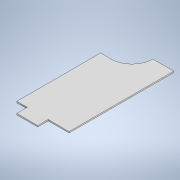
# Autodesk Inventor part: Rotation Board
Saved by Autodesk Inventor 2020 (Build 240168000, 168)
## iProperties
Created: 2021-02-27
Part Number: Rotation Board
Material: Generic
Document SubType Name: Modeling
Designer: tdmp4
Density: 1 g/cm^3
Appearance: Default
Author: tdmp4
Autodesk Inventor part; units mm, degrees
ref_plane "YZ Plane" through (0, 0, 0) normal (1, 0, 0) x (0, 1, 0)
ref_plane "XZ Plane" through (0, 0, 0) normal (0, 1, 0) x (-1, 0, 0)
ref_plane "XY Plane" through (0, 0, 0) normal (0, 0, 1) x (1, 0, 0)
sketch "Sketch1" plane through (0, 0, 0) normal (0, 1, 0) x (-1, 0, 0)
  line L0 (0, 0) -> (101.6, 0)
  line L1 (101.6, 0) -> (101.6, -254)
  line L2 (101.6, -254) -> (0, -254)
  line L3 (0, -254) -> (0, 0)
  dimension "d0" = 254
  dimension "d1" = 101.6
  constraints: 8 end point, 2 parallel, 1 horizontal, 1 perpendicular
  measures "d0" distance of L2.end L0.start
  measures "d1" distance of L0.start L0.end
extrude "Extrusion1" add sketch "Sketch1" along normal blind 3.175
sketch "Sketch2" plane through (-101.6, 0, 0) normal (0, 0, 1) x (1, 0, 0)
  line L0 (101.6, 3.175) -> (0, 3.175) projected
  line L1 (101.6, 0) -> (0, 0) projected
  line L2 (0, 3.175) -> (50.8, 3.175)
  line L3 (50.8, 3.175) -> (50.8, 0)
  line L4 (50.8, 0) -> (0, 0)
  line L5 (0, 0) -> (0, 3.175)
  constraints: 8 end point, 2 parallel, 1 horizontal, 1 midpoint, 1 perpendicular
extrude "Extrusion2" add sketch "Sketch2" along normal blind 25.4
sketch "Sketch3" plane through (0, 3.175, 0) normal (0, 1, 0) x (1, 0, 0)
  circle A0 centre (-101.6, 254) radius 50.8
  point P0 (0, 0)
  dimension "d6" = 101.6
  constraints: 1 centre point
  measures "d6" diameter of A0
extrude "Extrusion3" cut sketch "Sketch3" against normal blind 25.4
sketch "Sketch4" plane through (-101.6, 0, -203.2) normal (-1, 0, 0) x (0, 0, 1)
  line L0 (203.2, 3.175) -> (-50.8, 3.175) projected
  line L1 (203.2, 0) -> (-0.4173, 0)
  line L2 (-0.4173, 0) -> (-0.4173, 3.175)
  line L3 (-0.4173, 3.175) -> (203.2, 3.175)
  line L4 (203.2, 3.175) -> (203.2, 0)
  constraints: 8 end point, 2 parallel, 1 horizontal, 1 perpendicular, 1 point on line
extrude "Extrusion4" add sketch "Sketch4" along normal blind 25.4
body "Solid1"
